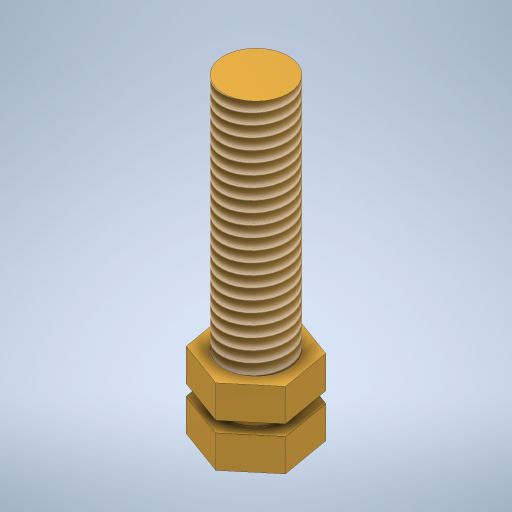
# Autodesk Inventor part: HUDOSN-1-54B
Saved by Autodesk Inventor 2024.2 (Build 282272000, 272)
## iProperties
Created: 2024-10-24
Part Number: HUDOSN-1-54B
Material: Generic
Document SubType Name: Modeling
Designer: Precisión-05
Density: 1 g/cm^3
Appearance: Default
Author: Precisión-05
Autodesk Inventor part; units mm, degrees
ref_plane "YZ Plane" through (0, 0, 0) normal (1, 0, 0) x (0, 1, 0)
ref_plane "XZ Plane" through (0, 0, 0) normal (0, 1, 0) x (-1, 0, 0)
ref_plane "XY Plane" through (0, 0, 0) normal (0, 0, 1) x (1, 0, 0)
sketch "Sketch1" plane through (0, 0, 0) normal (0, 0, 1) x (1, 0, 0)
  line L0 (-0.7879, 4.5) -> (3.5032, 2.9324)
  line L1 (3.5032, 2.9324) -> (4.2911, -1.5676)
  line L2 (4.2911, -1.5676) -> (0.7879, -4.5)
  line L3 (0.7879, -4.5) -> (-3.5032, -2.9324)
  line L4 (-3.5032, -2.9324) -> (-4.2911, 1.5676)
  line L5 (-4.2911, 1.5676) -> (-0.7879, 4.5)
  point P0 (0, 0)
  point P1 (0, 0)
  dimension "d0" = 9
  constraints: 12 end point, 1 coincident, 13 other
  measures "d0" vertical distance of L2.end L0.start
extrude "Extrusion1" add sketch "Sketch1" along normal blind 3
sketch "Sketch2" plane through (0, 0, 3) normal (0, 0, 1) x (1, 0, 0)
  circle A0 centre (0, 0) radius 3
  dimension "d3" = 6
  constraints: 1 centre point, 1 coincident
  measures "d3" diameter of A0
extrude "Extrusion2" add sketch "Sketch2" along normal blind 1
sketch "Sketch3" plane through (0, 0, 4) normal (0, 0, 1) x (1, 0, 0)
  line L0 (-0.7879, 4.5) -> (-4.2911, 1.5676) projected
  line L1 (-0.7879, 4.5) -> (3.5032, 2.9324)
  line L2 (3.5032, 2.9324) -> (4.2911, -1.5676)
  line L3 (4.2911, -1.5676) -> (0.7879, -4.5)
  line L4 (0.7879, -4.5) -> (-3.5032, -2.9324)
  line L5 (-3.5032, -2.9324) -> (-4.2911, 1.5676)
  line L6 (-4.2911, 1.5676) -> (-0.7879, 4.5)
  point P0 (0, 0)
  point P1 (0, 0)
  constraints: 12 end point, 1 coincident, 13 other
extrude "Extrusion3" add sketch "Sketch3" along normal blind 3
sketch "Sketch4" plane through (0, 0, 7) normal (0, 0, 1) x (1, 0, 0)
  circle A0 centre (0, 0) radius 3
  dimension "d8" = 6
  constraints: 1 centre point, 1 coincident
  measures "d8" diameter of A0
extrude "Extrusion4" add sketch "Sketch4" along normal blind 22
thread "Thread1" size "M6x1" class "6g" standard "ANSI Metric M Profile" full length
body "Solid1"
